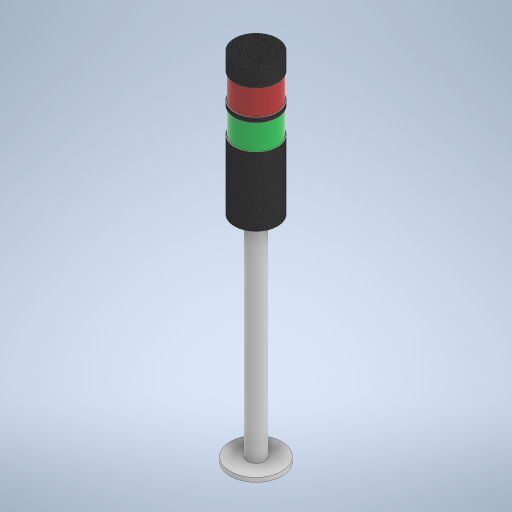
# Autodesk Inventor part: led
Saved by Autodesk Inventor 2023 (Build 270158000, 158)
## iProperties
Created: 2024-02-13
Part Number: led
Material: 일반
Document SubType Name: Modeling
Designer: ps737
Density: 1 g/cm^3
Appearance: 기본값
Author: ps737
Autodesk Inventor part; units mm, degrees
ref_plane "YZ Plane" through (0, 0, 0) normal (1, 0, 0) x (0, 1, 0)
ref_plane "XZ Plane" through (0, 0, 0) normal (0, 1, 0) x (-1, 0, 0)
ref_plane "XY Plane" through (0, 0, 0) normal (0, 0, 1) x (1, 0, 0)
sketch "스케치1" plane through (0, 0, 0) normal (0, 1, 0) x (-1, 0, 0)
  circle A0 centre (0, 0) radius 30
  circle A1 centre (0, 0) radius 10
  dimension "d0" = 60
  dimension "d1" = 20
  constraints: 2 centre point, 2 coincident
  measures "d0" diameter of A0
  measures "d1" diameter of A1
extrude "돌출1" add sketch "스케치1" along normal blind 5
extrude "돌출2" add sketch "스케치1" along normal blind 250 contours A1
sketch "스케치2" plane through (0, 250, 0) normal (0, 1, 0) x (1, 0, 0)
  circle A0 centre (0, 0) radius 25
  dimension "d6" = 50
  constraints: 1 centre point, 1 coincident
  measures "d6" diameter of A0
extrude "돌출3" add sketch "스케치2" along normal blind 80
sketch "스케치6" plane through (0, 330, 0) normal (0, 1, 0) x (1, 0, 0)
  circle A0 centre (0, 0) radius 25 projected
  circle A1 centre (0, 0) radius 24
  dimension "d15" = 48
  constraints: 1 centre point, 1 coincident
  measures "d15" diameter of A1
extrude "돌출6" add sketch "스케치6" along normal blind 30 contours A1
sketch "스케치7" plane through (0, 360, 0) normal (0, 1, 0) x (1, 0, 0)
  circle A0 centre (0, 0) radius 25
  dimension "d18" = 50
  constraints: 1 centre point, 1 coincident
  measures "d18" diameter of A0
extrude "돌출7" add sketch "스케치7" along normal blind 5
sketch "스케치8" plane through (0, 365, 0) normal (0, 1, 0) x (1, 0, 0)
  circle A0 centre (0, 0) radius 24
  dimension "d21" = 48
  constraints: 1 centre point, 1 coincident
  measures "d21" diameter of A0
extrude "돌출8" add sketch "스케치8" along normal blind 30
sketch "스케치9" plane through (0, 395, 0) normal (0, 1, 0) x (1, 0, 0)
  circle A0 centre (0, 0) radius 25
  dimension "d24" = 50
  constraints: 1 centre point, 1 coincident
  measures "d24" diameter of A0
extrude "돌출9" add sketch "스케치9" along normal blind 20
